Autodesk Inventor part; units mm, degrees
(part 2 of 8)
sketch "1" plane through (0, 0, 0) normal (0, 0, 1) x (1, 0, 0)
  arc A0 (47.7148, 33.2368) -> (47.5352, 33.0572) centre (47.625, 33.147) ccw
  arc A1 (30.9339, 69.4909) -> (31.1879, 69.4909) centre (31.0609, 69.4909) ccw
  line L0 (31.0609, 69.4909) -> (25.4, 63.83)
  arc A2 (25.3102, 63.9198) -> (25.4898, 63.7402) centre (25.4, 63.83) ccw
  line L1 (74.442, 14.6412) -> (67.4932, 21.59)
  arc A3 (46.228, 52.197) -> (46.228, 51.943) centre (46.228, 52.07) ccw
  arc A4 (52.451, 51.943) -> (52.451, 52.197) centre (52.451, 52.07) ccw
  line L2 (46.228, 52.07) -> (52.451, 52.07)
  arc A5 (55.1552, 71.891) -> (55.3348, 72.0706) centre (55.245, 71.9808) ccw
  arc A6 (55.3094, 72.096) -> (55.1298, 71.9164) centre (55.2196, 72.0062) ccw
  line L3 (55.245, 71.9808) -> (55.2196, 72.0062)
  arc A7 (55.118, 54.864) -> (55.372, 54.864) centre (55.245, 54.864) ccw
  arc A8 (55.372, 71.9808) -> (55.118, 71.9808) centre (55.245, 71.9808) ccw
  line L4 (55.245, 54.864) -> (55.245, 71.9808)
  arc A9 (52.3612, 52.1598) -> (52.5408, 51.9802) centre (52.451, 52.07) ccw
  arc A10 (55.3348, 54.7742) -> (55.1552, 54.9538) centre (55.245, 54.864) ccw
  line L5 (52.451, 52.07) -> (55.245, 54.864)
  arc A11 (30.3902, 36.4118) -> (30.5698, 36.2322) centre (30.48, 36.322) ccw
  arc A12 (46.3178, 51.9802) -> (46.1382, 52.1598) centre (46.228, 52.07) ccw
  line L6 (30.48, 36.322) -> (46.228, 52.07)
  arc A13 (31.1507, 69.4011) -> (30.9711, 69.5807) centre (31.0609, 69.4909) ccw
  line L7 (25.4, 36.322) -> (25.4, 63.83)
  arc A14 (25.527, 63.83) -> (25.273, 63.83) centre (25.4, 63.83) ccw
  arc A15 (25.273, 36.322) -> (25.527, 36.322) centre (25.4, 36.322) ccw
  arc A16 (53.9458, 80.9625) -> (53.9458, 81.5975) centre (53.9458, 81.28) ccw
  arc A17 (20.4098, 31.3318) -> (20.2302, 31.1522) centre (20.32, 31.242) ccw
  line L8 (74.442, 9.6412) -> (69.8808, 5.08)
  arc A18 (69.6563, 5.3045) -> (70.1053, 4.8555) centre (69.8808, 5.08) ccw
  arc A19 (74.6665, 9.4167) -> (74.2175, 9.8657) centre (74.442, 9.6412) ccw
  line L9 (57.4105, 5.08) -> (52.8493, 9.6412)
  arc A20 (53.0738, 9.8657) -> (52.6248, 9.4167) centre (52.8493, 9.6412) ccw
  arc A21 (57.186, 4.8555) -> (57.635, 5.3045) centre (57.4105, 5.08) ccw
  line L10 (69.8808, 5.08) -> (57.4105, 5.08)
  arc A22 (57.4105, 5.3975) -> (57.4105, 4.7625) centre (57.4105, 5.08) ccw
  arc A23 (69.8808, 4.7625) -> (69.8808, 5.3975) centre (69.8808, 5.08) ccw
  line L11 (52.8493, 9.6412) -> (48.2881, 5.08)
  arc A24 (48.0636, 5.3045) -> (48.5126, 4.8555) centre (48.2881, 5.08) ccw
  arc A25 (53.0738, 9.4167) -> (52.6248, 9.8657) centre (52.8493, 9.6412) ccw
  line L12 (48.2881, 5.08) -> (35.56, 5.08)
  line L13 (33.6795, 17.8825) -> (33.6795, 15.0888)
  arc A26 (33.5525, 15.0888) -> (33.8065, 15.0888) centre (33.6795, 15.0888) ccw
  arc A27 (33.8065, 17.8825) -> (33.5525, 17.8825) centre (33.6795, 17.8825) ccw
  line L14 (33.6796, 15.0886) -> (33.6795, 15.0888)
  arc A28 (33.7693, 15.1786) -> (33.5897, 14.999) centre (33.6795, 15.0888) ccw
  arc A29 (33.5898, 14.9988) -> (33.7694, 15.1784) centre (33.6796, 15.0886) ccw
  line L15 (33.6795, 17.8825) -> (20.32, 31.242)
  arc A30 (33.5897, 17.7927) -> (33.7693, 17.9723) centre (33.6795, 17.8825) ccw
  line L16 (20.32, 31.242) -> (20.32, 33.782)
  arc A31 (20.447, 33.782) -> (20.193, 33.782) centre (20.32, 33.782) ccw
  arc A32 (20.193, 31.242) -> (20.447, 31.242) centre (20.32, 31.242) ccw
  arc A33 (85.0002, 59.6002) -> (85.1798, 59.7798) centre (85.09, 59.69) ccw
  arc A34 (73.9474, 71.0122) -> (73.7678, 70.8326) centre (73.8576, 70.9224) ccw
  line L17 (85.09, 59.69) -> (73.8576, 70.9224)
  arc A35 (84.963, 50.8) -> (85.217, 50.8) centre (85.09, 50.8) ccw
  arc A36 (85.217, 59.69) -> (84.963, 59.69) centre (85.09, 59.69) ccw
  line L18 (85.09, 50.8) -> (85.09, 59.69)
  arc A37 (73.7306, 70.9224) -> (73.9846, 70.9224) centre (73.8576, 70.9224) ccw
  arc A38 (73.9846, 74.8321) -> (73.7306, 74.8321) centre (73.8576, 74.8321) ccw
  line L19 (73.8576, 70.9224) -> (73.8576, 74.8321)
  arc A39 (61.7944, 42.037) -> (61.7944, 41.783) centre (61.7944, 41.91) ccw
  arc A40 (76.2, 41.783) -> (76.2, 42.037) centre (76.2, 41.91) ccw
  line L20 (61.7944, 41.91) -> (76.2, 41.91)
  arc A41 (76.1102, 41.9998) -> (76.2898, 41.8202) centre (76.2, 41.91) ccw
  arc A42 (85.1798, 50.7102) -> (85.0002, 50.8898) centre (85.09, 50.8) ccw
  line L21 (76.2, 41.91) -> (85.09, 50.8)
  arc A43 (56.1166, 36.4118) -> (56.2962, 36.2322) centre (56.2064, 36.322) ccw
  arc A44 (61.8842, 41.8202) -> (61.7046, 41.9998) centre (61.7944, 41.91) ccw
  line L22 (56.2064, 36.322) -> (61.7944, 41.91)
  line L23 (27.94, 36.322) -> (27.94, 48.2127)
  arc A45 (28.067, 48.2127) -> (27.813, 48.2127) centre (27.94, 48.2127) ccw
  arc A46 (27.813, 36.322) -> (28.067, 36.322) centre (27.94, 36.322) ccw
  line L24 (27.94, 48.2127) -> (31.1842, 51.4569)
  arc A47 (31.274, 51.3671) -> (31.0944, 51.5467) centre (31.1842, 51.4569) ccw
  arc A48 (27.8502, 48.3025) -> (28.0298, 48.1229) centre (27.94, 48.2127) ccw
  arc A49 (69.4833, 56.5839) -> (69.4833, 56.3299) centre (69.4833, 56.4569) ccw
  arc A50 (74.3504, 56.3299) -> (74.3504, 56.5839) centre (74.3504, 56.4569) ccw
  line L25 (69.4833, 56.4569) -> (74.3504, 56.4569)
  arc A51 (50.9994, 36.322) -> (51.2534, 36.322) centre (51.1264, 36.322) ccw
  arc A52 (51.2534, 38.1) -> (50.9994, 38.1) centre (51.1264, 38.1) ccw
  line L26 (51.1264, 36.322) -> (51.1264, 38.1)
  arc A53 (69.5731, 56.3671) -> (69.3935, 56.5467) centre (69.4833, 56.4569) ccw
  arc A54 (51.0366, 38.1898) -> (51.2162, 38.0102) centre (51.1264, 38.1) ccw
  line L27 (69.4833, 56.4569) -> (51.1264, 38.1)
  arc A55 (53.5712, 36.322) -> (53.7617, 36.322) centre (53.6664, 36.322) ccw
  arc A56 (53.7617, 37.2029) -> (53.5712, 37.2029) centre (53.6664, 37.2029) ccw
  line L28 (53.6664, 36.322) -> (53.6664, 37.2029)
  arc A57 (70.5277, 53.9296) -> (70.393, 54.0643) centre (70.4604, 53.997) ccw
  arc A58 (53.599, 37.2703) -> (53.7338, 37.1356) centre (53.6664, 37.203) ccw
  line L29 (70.4604, 53.9969) -> (53.6664, 37.2029)
  arc A59 (76.8104, 53.9017) -> (76.8104, 54.0922) centre (76.8104, 53.9969) ccw
  arc A60 (70.4604, 54.0922) -> (70.4604, 53.9017) centre (70.4604, 53.9969) ccw
  line L30 (76.8104, 53.9969) -> (70.4604, 53.9969)
  arc A61 (79.283, 51.3896) -> (79.4177, 51.5243) centre (79.3503, 51.4569) ccw
  arc A62 (76.8777, 54.0643) -> (76.743, 53.9296) centre (76.8103, 53.997) ccw
  line L31 (79.3504, 51.4569) -> (76.8104, 53.9969)
  arc A63 (47.5352, 36.2848) -> (47.7148, 36.1052) centre (47.625, 36.195) ccw
  arc A64 (72.4798, 60.8702) -> (72.3002, 61.0498) centre (72.39, 60.96) ccw
  line L32 (47.625, 36.195) -> (72.39, 60.96)
  arc A65 (54.1744, 31.623) -> (54.1744, 31.877) centre (54.1744, 31.75) ccw
  arc A66 (49.022, 31.877) -> (49.022, 31.623) centre (49.022, 31.75) ccw
  line L33 (54.1744, 31.75) -> (49.022, 31.75)
  arc A67 (79.4774, 59.0796) -> (79.2234, 59.0796) centre (79.3504, 59.0796) ccw
  arc A68 (79.2234, 56.4569) -> (79.4774, 56.4569) centre (79.3504, 56.4569) ccw
  line L34 (79.3504, 59.0796) -> (79.3504, 56.4569)
  arc A69 (77.5598, 61.0498) -> (77.3802, 60.8702) centre (77.47, 60.96) ccw
  arc A70 (79.2606, 58.9898) -> (79.4402, 59.1694) centre (79.3504, 59.0796) ccw
  line L35 (77.47, 60.96) -> (79.3504, 59.0796)
  arc A71 (72.39, 61.087) -> (72.39, 60.833) centre (72.39, 60.96) ccw
  arc A72 (77.47, 60.833) -> (77.47, 61.087) centre (77.47, 60.96) ccw
  line L36 (72.39, 60.96) -> (77.47, 60.96)
  arc A73 (47.498, 33.147) -> (47.752, 33.147) centre (47.625, 33.147) ccw
  arc A74 (47.752, 36.195) -> (47.498, 36.195) centre (47.625, 36.195) ccw
  line L37 (47.625, 33.147) -> (47.625, 36.195)
  arc A75 (48.9322, 31.6602) -> (49.1118, 31.8398) centre (49.022, 31.75) ccw
  line L38 (27.94, 33.782) -> (27.94, 34.29)
  line L39 (49.022, 31.75) -> (47.625, 33.147)
  arc A76 (56.2962, 33.6922) -> (56.1166, 33.8718) centre (56.2064, 33.782) ccw
  arc A77 (54.0846, 31.8398) -> (54.2642, 31.6602) centre (54.1744, 31.75) ccw
  line L40 (56.2064, 33.782) -> (54.1744, 31.75)
  arc A78 (69.3639, 51.5839) -> (69.3639, 51.3299) centre (69.3639, 51.4569) ccw
  arc A79 (74.3504, 51.3299) -> (74.3504, 51.5839) centre (74.3504, 51.4569) ccw
  line L41 (69.3639, 51.4569) -> (74.3504, 51.4569)
  arc A80 (54.8504, 37.123) -> (55.03, 36.9434) centre (54.9402, 37.0332) ccw
  arc A81 (69.4537, 51.3671) -> (69.2741, 51.5467) centre (69.3639, 51.4569) ccw
  line L42 (54.9402, 37.0332) -> (69.3639, 51.4569)
  arc A82 (54.8132, 35.0558) -> (55.0672, 35.0558) centre (54.9402, 35.0558) ccw
  arc A83 (55.0672, 37.0332) -> (54.8132, 37.0332) centre (54.9402, 37.0332) ccw
  line L43 (54.9402, 35.0558) -> (54.9402, 37.0332)
  arc A84 (53.5766, 33.8718) -> (53.7562, 33.6922) centre (53.6664, 33.782) ccw
  arc A85 (55.03, 34.966) -> (54.8504, 35.1456) centre (54.9402, 35.0558) ccw
  line L44 (53.6664, 33.782) -> (54.9402, 35.0558)
  arc A86 (68.3984, 24.4475) -> (68.3984, 23.8125) centre (68.3984, 24.13) ccw
  arc A87 (75.8336, 23.8125) -> (75.8336, 24.4475) centre (75.8336, 24.13) ccw
  line L45 (68.3984, 24.13) -> (75.8336, 24.13)
  arc A88 (87.5979, 11.9167) -> (88.0469, 12.3657) centre (87.8224, 12.1412) ccw
  arc A89 (76.0581, 24.3545) -> (75.6091, 23.9055) centre (75.8336, 24.13) ccw
  line L46 (87.8224, 12.1412) -> (75.8336, 24.13)
  arc A90 (87.8224, 12.4587) -> (87.8224, 11.8237) centre (87.8224, 12.1412) ccw
  arc A91 (95.4424, 11.8237) -> (95.4424, 12.4587) centre (95.4424, 12.1412) ccw
  line L47 (87.8224, 12.1412) -> (95.4424, 12.1412)
  arc A92 (58.9709, 34.0065) -> (58.5219, 33.5575) centre (58.7464, 33.782) ccw
  arc A93 (68.1739, 23.9055) -> (68.6229, 24.3545) centre (68.3984, 24.13) ccw
  line L48 (58.7464, 33.782) -> (68.3984, 24.13)
  arc A94 (67.1284, 28.2575) -> (67.1284, 27.6225) centre (67.1284, 27.94) ccw
  arc A95 (90.5862, 27.6225) -> (90.5862, 28.2575) centre (90.5862, 27.94) ccw
  line L49 (67.1284, 27.94) -> (90.5862, 27.94)
  arc A96 (90.3616, 28.1645) -> (90.8107, 27.7155) centre (90.5862, 27.94) ccw
  arc A97 (95.6603, 32.5651) -> (95.2113, 33.0141) centre (95.4358, 32.7896) ccw
  line L50 (90.5862, 27.94) -> (95.4358, 32.7896)
  arc A98 (61.5109, 34.0065) -> (61.0619, 33.5575) centre (61.2864, 33.782) ccw
  arc A99 (66.9039, 27.7155) -> (67.3529, 28.1645) centre (67.1284, 27.94) ccw
  line L51 (61.2864, 33.782) -> (67.1284, 27.94)
  arc A100 (87.3125, 49.53) -> (87.9475, 49.53) centre (87.63, 49.53) ccw
  arc A101 (87.9475, 58.1297) -> (87.3125, 58.1297) centre (87.63, 58.1297) ccw
  line L52 (87.63, 49.53) -> (87.63, 58.1297)
  arc A102 (95.1249, 65.9421) -> (95.7599, 65.9421) centre (95.4424, 65.9421) ccw
  arc A103 (95.7599, 74.8321) -> (95.1249, 74.8321) centre (95.4424, 74.8321) ccw
  line L53 (95.4424, 65.9421) -> (95.4424, 74.8321)
  arc A104 (95.6669, 65.7176) -> (95.2179, 66.1666) centre (95.4424, 65.9421) ccw
  arc A105 (87.4055, 58.3542) -> (87.8545, 57.9052) centre (87.63, 58.1297) ccw
  line L54 (95.4424, 65.9421) -> (87.63, 58.1297)
  arc A106 (77.2455, 39.5945) -> (77.6945, 39.1455) centre (77.47, 39.37) ccw
  arc A107 (87.8545, 49.3055) -> (87.4055, 49.7545) centre (87.63, 49.53) ccw
  line L55 (77.47, 39.37) -> (87.63, 49.53)
  arc A108 (61.7944, 39.6875) -> (61.7944, 39.0525) centre (61.7944, 39.37) ccw
  arc A109 (77.47, 39.0525) -> (77.47, 39.6875) centre (77.47, 39.37) ccw
  line L56 (61.7944, 39.37) -> (77.47, 39.37)
  arc A110 (58.5219, 36.5465) -> (58.9709, 36.0975) centre (58.7464, 36.322) ccw
  arc A111 (28.067, 34.29) -> (27.813, 34.29) centre (27.94, 34.29) ccw
  arc A112 (27.813, 33.782) -> (28.067, 33.782) centre (27.94, 33.782) ccw
  line L57 (27.94, 34.29) -> (29.21, 35.56)
  arc A113 (29.2998, 35.4702) -> (29.1202, 35.6498) centre (29.21, 35.56) ccw
  arc A114 (27.8502, 34.3798) -> (28.0298, 34.2002) centre (27.94, 34.29) ccw
  line L58 (29.21, 44.4827) -> (36.1842, 51.4569)
  arc A115 (36.274, 51.3671) -> (36.0944, 51.5467) centre (36.1842, 51.4569) ccw
  arc A116 (29.1202, 44.5725) -> (29.2998, 44.3929) centre (29.21, 44.4827) ccw
  line L59 (29.21, 35.56) -> (29.21, 44.4827)
  arc A117 (29.337, 44.4827) -> (29.083, 44.4827) centre (29.21, 44.4827) ccw
  arc A118 (29.083, 35.56) -> (29.337, 35.56) centre (29.21, 35.56) ccw
  line L60 (12.085, 15.0469) -> (9.0831, 15.0469)
  arc A119 (9.0831, 15.1739) -> (9.0831, 14.9199) centre (9.0831, 15.0469) ccw
  arc A120 (12.085, 14.9199) -> (12.085, 15.1739) centre (12.085, 15.0469) ccw
  line L61 (9.0831, 15.0469) -> (5.08, 19.05)
  arc A121 (5.1698, 19.1398) -> (4.9902, 18.9602) centre (5.08, 19.05) ccw
  arc A122 (8.9933, 14.9571) -> (9.1729, 15.1367) centre (9.0831, 15.0469) ccw
  line L62 (5.08, 19.05) -> (5.08, 26.67)
  arc A123 (5.207, 26.67) -> (4.953, 26.67) centre (5.08, 26.67) ccw
  arc A124 (4.953, 19.05) -> (5.207, 19.05) centre (5.08, 19.05) ccw
  line L63 (7.62, 29.21) -> (5.08, 26.67)
  arc A125 (4.9902, 26.7598) -> (5.1698, 26.5802) centre (5.08, 26.67) ccw
  arc A126 (7.7098, 29.1202) -> (7.5302, 29.2998) centre (7.62, 29.21) ccw
  line L64 (15.24, 33.782) -> (10.668, 29.21)
  arc A127 (10.5782, 29.2998) -> (10.7578, 29.1202) centre (10.668, 29.21) ccw
  arc A128 (15.3298, 33.6922) -> (15.1502, 33.8718) centre (15.24, 33.782) ccw
  line L65 (10.668, 29.21) -> (7.62, 29.21)
  arc A129 (7.62, 29.337) -> (7.62, 29.083) centre (7.62, 29.21) ccw
  arc A130 (10.668, 29.083) -> (10.668, 29.337) centre (10.668, 29.21) ccw
  line L66 (17.78, 33.782) -> (19.05, 35.052)
  arc A131 (19.1398, 34.9622) -> (18.9602, 35.1418) centre (19.05, 35.052) ccw
  arc A132 (21.463, 33.147) -> (21.717, 33.147) centre (21.59, 33.147) ccw
  arc A133 (17.6902, 33.8718) -> (17.8698, 33.6922) centre (17.78, 33.782) ccw
  line L67 (19.05, 59.7948) -> (12.0927, 66.7521)
  arc A134 (12.1825, 66.8419) -> (12.0029, 66.6623) centre (12.0927, 66.7521) ccw
  arc A135 (18.9602, 59.705) -> (19.1398, 59.8846) centre (19.05, 59.7948) ccw
  line L68 (12.0927, 66.7521) -> (12.0927, 71.8321)
  arc A136 (12.2197, 71.8321) -> (11.9657, 71.8321) centre (12.0927, 71.8321) ccw
  arc A137 (11.9657, 66.7521) -> (12.2197, 66.7521) centre (12.0927, 66.7521) ccw
  line L69 (19.05, 35.052) -> (19.05, 59.7948)
  arc A138 (19.177, 59.7948) -> (18.923, 59.7948) centre (19.05, 59.7948) ccw
  arc A139 (18.923, 35.052) -> (19.177, 35.052) centre (19.05, 35.052) ccw
  line L70 (58.7464, 36.322) -> (61.7944, 39.37)
  arc A140 (35.56, 5.3975) -> (35.56, 4.7625) centre (35.56, 5.08) ccw
  arc A141 (48.2881, 4.7625) -> (48.2881, 5.3975) centre (48.2881, 5.08) ccw
  line L71 (35.56, 5.08) -> (30.6796, 9.9604)
  arc A142 (30.9041, 10.1849) -> (30.4551, 9.7359) centre (30.6796, 9.9604) ccw
  arc A143 (35.3355, 4.8555) -> (35.7845, 5.3045) centre (35.56, 5.08) ccw
  line L72 (30.6796, 9.9604) -> (30.6796, 10.0886)
  arc A144 (30.9971, 10.0886) -> (30.3621, 10.0886) centre (30.6796, 10.0886) ccw
  arc A145 (30.3621, 9.9604) -> (30.9971, 9.9604) centre (30.6796, 9.9604) ccw
  line L73 (30.6796, 10.0886) -> (25.671, 5.08)
  arc A146 (25.4465, 5.3045) -> (25.8955, 4.8555) centre (25.671, 5.08) ccw
  arc A147 (30.9041, 9.8641) -> (30.4551, 10.3131) centre (30.6796, 10.0886) ccw
  line L74 (15.0927, 76.8321) -> (19.5406, 81.28)
  arc A148 (19.7651, 81.0555) -> (19.3161, 81.5045) centre (19.5406, 81.28) ccw
  arc A149 (14.8682, 77.0566) -> (15.3172, 76.6076) centre (15.0927, 76.8321) ccw
  line L75 (14.0519, 5.08) -> (9.085, 10.0469)
  arc A150 (9.3095, 10.2714) -> (8.8605, 9.8224) centre (9.085, 10.0469) ccw
  arc A151 (13.8274, 4.8555) -> (14.2764, 5.3045) centre (14.0519, 5.08) ccw
  line L76 (25.671, 5.08) -> (14.0519, 5.08)
  arc A152 (14.0519, 5.3975) -> (14.0519, 4.7625) centre (14.0519, 5.08) ccw
  arc A153 (25.671, 4.7625) -> (25.671, 5.3975) centre (25.671, 5.08) ccw
  line L77 (48.641, 25.4) -> (48.641, 27.559)
  arc A154 (48.9585, 27.559) -> (48.3235, 27.559) centre (48.641, 27.559) ccw
  arc A155 (48.3235, 25.4) -> (48.9585, 25.4) centre (48.641, 25.4) ccw
  line L78 (39.878, 36.322) -> (35.56, 36.322)
  arc A156 (35.56, 36.6395) -> (35.56, 36.0045) centre (35.56, 36.322) ccw
  arc A157 (39.878, 36.0045) -> (39.878, 36.6395) centre (39.878, 36.322) ccw
  line L79 (48.641, 27.559) -> (39.878, 36.322)
  arc A158 (40.1025, 36.5465) -> (39.6535, 36.0975) centre (39.878, 36.322) ccw
  arc A159 (48.4165, 27.3345) -> (48.8655, 27.7835) centre (48.641, 27.559) ccw
  arc A160 (62.0189, 39.1455) -> (61.5699, 39.5945) centre (61.7944, 39.37) ccw
  line L80 (9.085, 10.0469) -> (3.175, 15.9569)
  arc A161 (74.2175, 14.4167) -> (74.6665, 14.8657) centre (74.442, 14.6412) ccw
  line L81 (41.275, 21.59) -> (30.48, 32.385)
  arc A162 (30.7045, 32.6095) -> (30.2555, 32.1605) centre (30.48, 32.385) ccw
  arc A163 (41.0505, 21.3655) -> (41.4995, 21.8145) centre (41.275, 21.59) ccw
  line L82 (30.48, 32.385) -> (30.48, 33.782)
  arc A164 (30.7975, 33.782) -> (30.1625, 33.782) centre (30.48, 33.782) ccw
  arc A165 (30.1625, 32.385) -> (30.7975, 32.385) centre (30.48, 32.385) ccw
  line L83 (67.4932, 21.59) -> (41.275, 21.59)
  arc A166 (41.275, 21.9075) -> (41.275, 21.2725) centre (41.275, 21.59) ccw
  arc A167 (67.4932, 21.2725) -> (67.4932, 21.9075) centre (67.4932, 21.59) ccw
  line L84 (33.02, 36.322) -> (47.5751, 50.8771)
  arc A168 (47.6649, 50.7873) -> (47.4853, 50.9669) centre (47.5751, 50.8771) ccw
  arc A169 (32.9302, 36.4118) -> (33.1098, 36.2322) centre (33.02, 36.322) ccw
  line L85 (47.5751, 50.8771) -> (55.2831, 50.8771)
  arc A170 (55.2831, 50.7501) -> (55.2831, 51.0041) centre (55.2831, 50.8771) ccw
  arc A171 (47.5751, 51.0041) -> (47.5751, 50.7501) centre (47.5751, 50.8771) ccw
  line L86 (52.8493, 14.6412) -> (42.5088, 14.6412)
  arc A172 (42.5088, 14.7682) -> (42.5088, 14.5142) centre (42.5088, 14.6412) ccw
  arc A173 (52.8493, 14.5142) -> (52.8493, 14.7682) centre (52.8493, 14.6412) ccw
  line L87 (42.5088, 14.6412) -> (24.13, 33.02)
  arc A174 (24.2198, 33.1098) -> (24.0402, 32.9302) centre (24.13, 33.02) ccw
  arc A175 (42.419, 14.5514) -> (42.5986, 14.731) centre (42.5088, 14.6412) ccw
  line L88 (24.13, 35.052) -> (22.86, 36.322)
  arc A176 (22.9498, 36.4118) -> (22.7702, 36.2322) centre (22.86, 36.322) ccw
  arc A177 (24.0402, 34.9622) -> (24.2198, 35.1418) centre (24.13, 35.052) ccw
  line L89 (24.13, 33.02) -> (24.13, 35.052)
  arc A178 (24.257, 35.052) -> (24.003, 35.052) centre (24.13, 35.052) ccw
  arc A179 (24.003, 33.02) -> (24.257, 33.02) centre (24.13, 33.02) ccw
  line L90 (57.8493, 14.6412) -> (55.3493, 12.1412)
  arc A180 (55.2595, 12.231) -> (55.4391, 12.0514) centre (55.3493, 12.1412) ccw
  arc A181 (57.9391, 14.5514) -> (57.7595, 14.731) centre (57.8493, 14.6412) ccw
  line L91 (21.59, 35.052) -> (20.32, 36.322)
  arc A182 (20.4098, 36.4118) -> (20.2302, 36.2322) centre (20.32, 36.322) ccw
  arc A183 (21.5002, 34.9622) -> (21.6798, 35.1418) centre (21.59, 35.052) ccw
  line L92 (55.3493, 12.1412) -> (42.5958, 12.1412)
  arc A184 (42.5958, 12.2365) -> (42.5958, 12.046) centre (42.5958, 12.1413) ccw
  arc A185 (55.3493, 12.046) -> (55.3493, 12.2365) centre (55.3493, 12.1413) ccw
  line L93 (42.5958, 12.1412) -> (21.59, 33.147)
  arc A186 (21.6798, 33.2368) -> (21.5002, 33.0572) centre (21.59, 33.147) ccw
  arc A187 (42.506, 12.0514) -> (42.6856, 12.231) centre (42.5958, 12.1412) ccw
  line L94 (21.59, 33.147) -> (21.59, 35.052)
  arc A188 (21.717, 35.052) -> (21.463, 35.052) centre (21.59, 35.052) ccw
  arc A189 (3.3995, 16.1814) -> (2.9505, 15.7324) centre (3.175, 15.9569) ccw
  arc A190 (8.8605, 9.8224) -> (9.3095, 10.2714) centre (9.085, 10.0469) ccw
  line L95 (3.175, 78.105) -> (6.35, 81.28)
  arc A191 (6.5745, 81.0555) -> (6.1255, 81.5045) centre (6.35, 81.28) ccw
  arc A192 (2.9505, 78.3295) -> (3.3995, 77.8805) centre (3.175, 78.105) ccw
  line L96 (6.35, 81.28) -> (10.6448, 81.28)
  arc A193 (10.6448, 80.9625) -> (10.6448, 81.5975) centre (10.6448, 81.28) ccw
  arc A194 (6.35, 81.5975) -> (6.35, 80.9625) centre (6.35, 81.28) ccw
  line L97 (10.6448, 81.28) -> (15.0927, 76.8321)
  arc A195 (14.8682, 76.6076) -> (15.3172, 77.0566) centre (15.0927, 76.8321) ccw
  arc A196 (10.8693, 81.5045) -> (10.4203, 81.0555) centre (10.6448, 81.28) ccw
  line L98 (3.175, 15.9569) -> (3.175, 78.105)
  arc A197 (3.4925, 78.105) -> (2.8575, 78.105) centre (3.175, 78.105) ccw
  arc A198 (2.8575, 15.9569) -> (3.4925, 15.9569) centre (3.175, 15.9569) ccw
  line L99 (53.9458, 81.28) -> (58.2196, 77.0062)
  arc A199 (57.9951, 76.7817) -> (58.4441, 77.2307) centre (58.2196, 77.0062) ccw
  arc A200 (54.1703, 81.5045) -> (53.7213, 81.0555) centre (53.9458, 81.28) ccw
  line L100 (60.8231, 74.4027) -> (60.8231, 58.4171)
  arc A201 (60.5056, 58.4171) -> (61.1406, 58.4171) centre (60.8231, 58.4171) ccw
  arc A202 (61.1406, 74.4027) -> (60.5056, 74.4027) centre (60.8231, 74.4027) ccw
  line L101 (58.2831, 55.8771) -> (60.8231, 58.4171)
  arc A203 (61.0476, 58.1926) -> (60.5986, 58.6416) centre (60.8231, 58.4171) ccw
  arc A204 (58.0586, 56.1016) -> (58.5076, 55.6526) centre (58.2831, 55.8771) ccw
  line L102 (60.8231, 74.4027) -> (58.2196, 77.0062)
  arc A205 (58.4441, 77.2307) -> (57.9951, 76.7817) centre (58.2196, 77.0062) ccw
  arc A206 (60.5986, 74.1782) -> (61.0476, 74.6272) centre (60.8231, 74.4027) ccw
  line L103 (19.5406, 81.28) -> (53.9458, 81.28)
  arc A207 (19.5406, 81.5975) -> (19.5406, 80.9625) centre (19.5406, 81.28) ccw
  line L104 (52.2831, 55.8771) -> (47.2002, 60.96)
  arc A208 (47.4247, 61.1845) -> (46.9757, 60.7355) centre (47.2002, 60.96) ccw
  arc A209 (52.0586, 55.6526) -> (52.5076, 56.1016) centre (52.2831, 55.8771) ccw
  line L105 (47.2002, 60.96) -> (35.56, 60.96)
  arc A210 (35.56, 61.2775) -> (35.56, 60.6425) centre (35.56, 60.96) ccw
  arc A211 (47.2002, 60.6425) -> (47.2002, 61.2775) centre (47.2002, 60.96) ccw
  line L106 (31.1842, 56.4569) -> (31.1842, 56.5842)
  arc A212 (31.5017, 56.5842) -> (30.8667, 56.5842) centre (31.1842, 56.5842) ccw
  arc A213 (30.8667, 56.4569) -> (31.5017, 56.4569) centre (31.1842, 56.4569) ccw
  line L107 (35.56, 60.96) -> (31.1842, 56.5842)
  arc A214 (30.9597, 56.8087) -> (31.4087, 56.3597) centre (31.1842, 56.5842) ccw
  arc A215 (35.7845, 60.7355) -> (35.3355, 61.1845) centre (35.56, 60.96) ccw
  arc A216 (67.7177, 21.8145) -> (67.2687, 21.3655) centre (67.4932, 21.59) ccw
  line L108 (25.4, 33.782) -> (26.67, 35.052)
  arc A217 (26.7598, 34.9622) -> (26.5802, 35.1418) centre (26.67, 35.052) ccw
  arc A218 (25.3102, 33.8718) -> (25.4898, 33.6922) centre (25.4, 33.782) ccw
  line L109 (26.67, 63.021) -> (36.0609, 72.4119)
  arc A219 (36.1507, 72.3221) -> (35.9711, 72.5017) centre (36.0609, 72.4119) ccw
  arc A220 (26.5802, 63.1108) -> (26.7598, 62.9312) centre (26.67, 63.021) ccw
  line L110 (26.67, 35.052) -> (26.67, 63.021)
  arc A221 (26.797, 63.021) -> (26.543, 63.021) centre (26.67, 63.021) ccw
  arc A222 (26.543, 35.052) -> (26.797, 35.052) centre (26.67, 35.052) ccw
  line L111 (31.0609, 69.4909) -> (31.0609, 72.4119)
  arc A223 (31.1879, 72.4119) -> (30.9339, 72.4119) centre (31.0609, 72.4119) ccw
  constraints: 613 point on circle, 224 centre point, 224 end point, 6 point on line
sketch "16" plane through (0, 0, 0) normal (0, 0, 1) x (1, 0, 0)
  line L0 (52.2196, 77.0062) -> (47.9458, 81.28)
  arc A0 (56.4934, 81.5975) -> (56.4934, 80.9625) centre (56.4934, 81.28) ccw
  arc A1 (73.4097, 80.9625) -> (73.4097, 81.5975) centre (73.4097, 81.28) ccw
  arc A2 (7.493, 25.4) -> (7.747, 25.4) centre (7.62, 25.4) ccw
  arc A3 (7.747, 33.782) -> (7.493, 33.782) centre (7.62, 33.782) ccw
  line L1 (7.62, 25.4) -> (7.62, 33.782)
  arc A4 (13.843, 31.75) -> (14.097, 31.75) centre (13.97, 31.75) ccw
  arc A5 (14.097, 35.052) -> (13.843, 35.052) centre (13.97, 35.052) ccw
  line L2 (13.97, 31.75) -> (13.97, 35.052)
  arc A6 (13.8802, 34.9622) -> (14.0598, 35.1418) centre (13.97, 35.052) ccw
  arc A7 (12.7898, 36.4118) -> (12.6102, 36.2322) centre (12.7, 36.322) ccw
  line L3 (13.97, 35.052) -> (12.7, 36.322)
  arc A8 (20.2302, 25.3102) -> (20.4098, 25.4898) centre (20.32, 25.4) ccw
  arc A9 (14.0598, 31.8398) -> (13.8802, 31.6602) centre (13.97, 31.75) ccw
  line L4 (20.32, 25.4) -> (13.97, 31.75)
  arc A10 (22.733, 25.4) -> (22.987, 25.4) centre (22.86, 25.4) ccw
  arc A11 (22.987, 33.782) -> (22.733, 33.782) centre (22.86, 33.782) ccw
  line L5 (22.86, 25.4) -> (22.86, 33.782)
  arc A12 (11.303, 29.21) -> (11.557, 29.21) centre (11.43, 29.21) ccw
  arc A13 (11.557, 35.052) -> (11.303, 35.052) centre (11.43, 35.052) ccw
  line L6 (11.43, 29.21) -> (11.43, 35.052)
  arc A14 (11.3402, 34.9622) -> (11.5198, 35.1418) centre (11.43, 35.052) ccw
  arc A15 (10.2498, 36.4118) -> (10.0702, 36.2322) centre (10.16, 36.322) ccw
  line L7 (11.43, 35.052) -> (10.16, 36.322)
  arc A16 (15.1502, 25.3102) -> (15.3298, 25.4898) centre (15.24, 25.4) ccw
  arc A17 (11.5198, 29.2998) -> (11.3402, 29.1202) centre (11.43, 29.21) ccw
  line L8 (15.24, 25.4) -> (11.43, 29.21)
  arc A18 (12.573, 30.48) -> (12.827, 30.48) centre (12.7, 30.48) ccw
  arc A19 (12.827, 33.782) -> (12.573, 33.782) centre (12.7, 33.782) ccw
  line L9 (12.7, 30.48) -> (12.7, 33.782)
  arc A20 (17.6902, 25.3102) -> (17.8698, 25.4898) centre (17.78, 25.4) ccw
  arc A21 (12.7898, 30.5698) -> (12.6102, 30.3902) centre (12.7, 30.48) ccw
  line L10 (17.78, 25.4) -> (12.7, 30.48)
  arc A22 (10.033, 27.94) -> (10.287, 27.94) centre (10.16, 27.94) ccw
  arc A23 (10.287, 33.782) -> (10.033, 33.782) centre (10.16, 33.782) ccw
  line L11 (10.16, 27.94) -> (10.16, 33.782)
  arc A24 (12.6102, 25.3102) -> (12.7898, 25.4898) centre (12.7, 25.4) ccw
  arc A25 (10.2498, 28.0298) -> (10.0702, 27.8502) centre (10.16, 27.94) ccw
  line L12 (12.7, 25.4) -> (10.16, 27.94)
  line L13 (19.1328, 55.7972) -> (17.0355, 55.7972)
  line L14 (56.4934, 81.28) -> (73.4097, 81.28)
  arc A26 (51.9951, 77.2307) -> (52.4441, 76.7817) centre (52.2196, 77.0062) ccw
  arc A27 (56.7179, 81.0555) -> (56.2689, 81.5045) centre (56.4934, 81.28) ccw
  line L15 (52.2196, 77.0062) -> (56.4934, 81.28)
  arc A28 (30.8364, 77.2394) -> (31.2854, 77.6884) centre (31.0609, 77.4639) ccw
  arc A29 (27.4693, 81.5045) -> (27.0203, 81.0555) centre (27.2448, 81.28) ccw
  line L16 (31.0609, 77.4639) -> (27.2448, 81.28)
  arc A30 (30.7434, 77.4119) -> (31.3784, 77.4119) centre (31.0609, 77.4119) ccw
  arc A31 (31.3784, 77.4639) -> (30.7434, 77.4639) centre (31.0609, 77.4639) ccw
  line L17 (31.0609, 77.4119) -> (31.0609, 77.4639)
  arc A32 (35.2209, 81.28) -> (34.5859, 81.28) centre (34.9034, 81.28) ccw
  arc A33 (34.5859, 81.2544) -> (35.2209, 81.2544) centre (34.9034, 81.2544) ccw
  line L18 (34.9034, 81.28) -> (34.9034, 81.2544)
  arc A34 (30.8364, 77.6364) -> (31.2854, 77.1874) centre (31.0609, 77.4119) ccw
  arc A35 (35.1279, 81.0299) -> (34.6789, 81.4789) centre (34.9034, 81.2544) ccw
  line L19 (31.0609, 77.4119) -> (34.9034, 81.2544)
  arc A36 (44.9875, 21.3655) -> (45.4365, 21.8145) centre (45.212, 21.59) ccw
  arc A37 (33.2445, 34.0065) -> (32.7955, 33.5575) centre (33.02, 33.782) ccw
  line L20 (45.212, 21.59) -> (33.02, 33.782)
  arc A38 (50.8, 21.2725) -> (50.8, 21.9075) centre (50.8, 21.59) ccw
  arc A39 (45.212, 21.9075) -> (45.212, 21.2725) centre (45.212, 21.59) ccw
  arc A40 (53.9455, 24.2865) -> (53.4965, 24.7355) centre (53.721, 24.511) ccw
  arc A41 (50.5755, 21.8145) -> (51.0245, 21.3655) centre (50.8, 21.59) ccw
  line L21 (53.721, 24.511) -> (50.8, 21.59)
  arc A42 (54.0385, 25.4) -> (53.4035, 25.4) centre (53.721, 25.4) ccw
  arc A43 (53.4035, 24.511) -> (54.0385, 24.511) centre (53.721, 24.511) ccw
  line L22 (53.721, 25.4) -> (53.721, 24.511)
  arc A44 (64.3639, 25.6245) -> (64.8129, 25.1755) centre (64.5884, 25.4) ccw
  arc A45 (68.6229, 28.9855) -> (68.1739, 29.4345) centre (68.3984, 29.21) ccw
  line L23 (64.5884, 25.4) -> (68.3984, 29.21)
  arc A46 (56.261, 25.7175) -> (56.261, 25.0825) centre (56.261, 25.4) ccw
  arc A47 (64.5884, 25.0825) -> (64.5884, 25.7175) centre (64.5884, 25.4) ccw
  line L24 (56.261, 25.4) -> (64.5884, 25.4)
  arc A48 (56.261, 25.0825) -> (56.261, 25.7175) centre (56.261, 25.4) ccw
  arc A49 (53.721, 25.7175) -> (53.721, 25.0825) centre (53.721, 25.4) ccw
  line L25 (56.261, 25.4) -> (53.721, 25.4)
  arc A50 (20.0519, 5.3975) -> (20.0519, 4.7625) centre (20.0519, 5.08) ccw
  arc A51 (31.6981, 4.7625) -> (31.6981, 5.3975) centre (31.6981, 5.08) ccw
  line L26 (20.0519, 5.08) -> (31.6981, 5.08)
  arc A52 (15.3095, 10.2714) -> (14.8605, 9.8224) centre (15.085, 10.0469) ccw
  arc A53 (19.8274, 4.8555) -> (20.2764, 5.3045) centre (20.0519, 5.08) ccw
  line L27 (15.085, 10.0469) -> (20.0519, 5.08)
  arc A54 (8.8232, 55.5727) -> (9.2722, 56.0217) centre (9.0477, 55.7972) ccw
  arc A55 (8.0022, 57.2917) -> (7.5532, 56.8427) centre (7.7777, 57.0672) ccw
  line L28 (9.0477, 55.7972) -> (7.7777, 57.0672)
  arc A56 (73.9775, 28.8925) -> (73.9775, 29.5275) centre (73.9775, 29.21) ccw
  arc A57 (68.3984, 29.5275) -> (68.3984, 28.8925) centre (68.3984, 29.21) ccw
  line L29 (73.9775, 29.21) -> (68.3984, 29.21)
  arc A58 (68.1739, 28.9855) -> (68.6229, 29.4345) centre (68.3984, 29.21) ccw
  arc A59 (61.5109, 36.5465) -> (61.0619, 36.0975) centre (61.2864, 36.322) ccw
  line L30 (68.3984, 29.21) -> (61.2864, 36.322)
  arc A60 (80.2345, 35.018) -> (79.7855, 35.467) centre (80.01, 35.2425) ccw
  arc A61 (73.753, 29.4345) -> (74.202, 28.9855) centre (73.9775, 29.21) ccw
  line L31 (80.01, 35.2425) -> (73.9775, 29.21)
  arc A62 (31.3806, 5.08) -> (32.0156, 5.08) centre (31.6981, 5.08) ccw
  arc A63 (32.0156, 5.1071) -> (31.3806, 5.1071) centre (31.6981, 5.1071) ccw
  line L32 (31.6981, 5.08) -> (31.6981, 5.1071)
  arc A64 (36.9041, 9.8641) -> (36.4551, 10.3131) centre (36.6796, 10.0886) ccw
  arc A65 (31.4736, 5.3316) -> (31.9226, 4.8826) centre (31.6981, 5.1071) ccw
  line L33 (36.6796, 10.0886) -> (31.6981, 5.1071)
  arc A66 (41.4637, 4.8555) -> (41.9127, 5.3045) centre (41.6882, 5.08) ccw
  arc A67 (36.9041, 10.3131) -> (36.4551, 9.8641) centre (36.6796, 10.0886) ccw
  line L34 (41.6882, 5.08) -> (36.6796, 10.0886)
  arc A68 (53.2935, 4.7625) -> (53.2935, 5.3975) centre (53.2935, 5.08) ccw
  arc A69 (41.6882, 5.3975) -> (41.6882, 4.7625) centre (41.6882, 5.08) ccw
  line L35 (53.2935, 5.08) -> (41.6882, 5.08)
  arc A70 (58.0738, 9.4113) -> (57.6248, 9.8603) centre (57.8493, 9.6358) ccw
  arc A71 (53.069, 5.3045) -> (53.518, 4.8555) centre (53.2935, 5.08) ccw
  line L36 (57.8493, 9.6358) -> (53.2935, 5.08)
  arc A72 (58.1668, 9.6412) -> (57.5318, 9.6412) centre (57.8493, 9.6412) ccw
  arc A73 (57.5318, 9.6358) -> (58.1668, 9.6358) centre (57.8493, 9.6358) ccw
  line L37 (57.8493, 9.6412) -> (57.8493, 9.6358)
  arc A74 (74.8808, 4.7625) -> (74.8808, 5.3975) centre (74.8808, 5.08) ccw
  line L38 (50.8, 21.59) -> (45.212, 21.59)
  arc A75 (16.811, 55.5727) -> (17.26, 56.0217) centre (17.0355, 55.7972) ccw
  arc A76 (15.2722, 58.0095) -> (14.8232, 57.5605) centre (15.0477, 57.785) ccw
  line L39 (17.0355, 55.7972) -> (15.0477, 57.785)
  arc A77 (17.0355, 55.4797) -> (17.0355, 56.1147) centre (17.0355, 55.7972) ccw
  arc A78 (15.0477, 56.1147) -> (15.0477, 55.4797) centre (15.0477, 55.7972) ccw
  line L40 (17.0355, 55.7972) -> (15.0477, 55.7972)
  arc A79 (19.1328, 55.4797) -> (19.1328, 56.1147) centre (19.1328, 55.7972) ccw
  arc A80 (17.0355, 56.1147) -> (17.0355, 55.4797) centre (17.0355, 55.7972) ccw
  arc A81 (95.4424, 53.3219) -> (95.4424, 54.5919) centre (95.4424, 53.9569) ccw
  arc A82 (35.3355, 39.1455) -> (35.7845, 39.5945) centre (35.56, 39.37) ccw
  arc A83 (19.3573, 56.0217) -> (18.9083, 55.5727) centre (19.1328, 55.7972) ccw
  line L41 (35.56, 39.37) -> (19.1328, 55.7972)
  arc A84 (35.2425, 36.322) -> (35.8775, 36.322) centre (35.56, 36.322) ccw
  arc A85 (35.8775, 39.37) -> (35.2425, 39.37) centre (35.56, 39.37) ccw
  line L42 (35.56, 36.322) -> (35.56, 39.37)
  arc A86 (14.8232, 77.0116) -> (15.2722, 76.5625) centre (15.0477, 76.787) ccw
  arc A87 (15.3172, 76.6076) -> (14.8682, 77.0566) centre (15.0927, 76.8321) ccw
  line L43 (15.0477, 76.7871) -> (15.0927, 76.8321)
  arc A88 (14.7302, 57.785) -> (15.3652, 57.785) centre (15.0477, 57.785) ccw
  arc A89 (15.3652, 76.7871) -> (14.7302, 76.7871) centre (15.0477, 76.7871) ccw
  line L44 (15.0477, 57.785) -> (15.0477, 76.7871)
  arc A90 (14.7302, 55.7972) -> (15.3652, 55.7972) centre (15.0477, 55.7972) ccw
  arc A91 (15.3652, 57.785) -> (14.7302, 57.785) centre (15.0477, 57.785) ccw
  line L45 (15.0477, 55.7972) -> (15.0477, 57.785)
  arc A92 (8.763, 26.67) -> (9.017, 26.67) centre (8.89, 26.67) ccw
  arc A93 (9.017, 35.052) -> (8.763, 35.052) centre (8.89, 35.052) ccw
  line L46 (8.89, 26.67) -> (8.89, 35.052)
  arc A94 (8.8002, 34.9622) -> (8.9798, 35.1418) centre (8.89, 35.052) ccw
  arc A95 (7.7098, 36.4118) -> (7.5302, 36.2322) centre (7.62, 36.322) ccw
  line L47 (8.89, 35.052) -> (7.62, 36.322)
  arc A96 (10.0702, 25.3102) -> (10.2498, 25.4898) centre (10.16, 25.4) ccw
  arc A97 (8.9798, 26.7598) -> (8.8002, 26.5802) centre (8.89, 26.67) ccw
  line L48 (10.16, 25.4) -> (8.89, 26.67)
  arc A98 (11.7302, 39.5143) -> (12.3652, 39.5143) centre (12.0477, 39.5143) ccw
  arc A99 (12.3652, 50.7972) -> (11.7302, 50.7972) centre (12.0477, 50.7972) ccw
  line L49 (12.0477, 39.5143) -> (12.0477, 50.7972)
  arc A100 (15.0155, 36.0975) -> (15.4645, 36.5465) centre (15.24, 36.322) ccw
  arc A101 (12.2722, 39.7388) -> (11.8232, 39.2898) centre (12.0477, 39.5143) ccw
  line L50 (15.24, 36.322) -> (12.0477, 39.5143)
  arc A102 (82.2789, 35.6915) -> (83.177, 34.7935) centre (82.728, 35.2425) ccw
  arc A103 (101.8848, 53.5013) -> (100.9868, 54.3993) centre (101.4358, 53.9503) ccw
  line L51 (82.728, 35.2425) -> (101.4358, 53.9503)
  arc A104 (40.3225, 38.862) -> (40.9575, 38.862) centre (40.64, 38.862) ccw
  arc A105 (40.9575, 72.8328) -> (40.3225, 72.8328) centre (40.64, 72.8328) ccw
  line L52 (40.64, 38.862) -> (40.64, 72.8328)
  arc A106 (40.4155, 72.6083) -> (40.8645, 73.0573) centre (40.64, 72.8328) ccw
  arc A107 (36.2854, 77.6364) -> (35.8364, 77.1874) centre (36.0609, 77.4119) ccw
  line L53 (40.64, 72.8328) -> (36.0609, 77.4119)
  arc A108 (35.3355, 34.0065) -> (35.7845, 33.5575) centre (35.56, 33.782) ccw
  arc A109 (40.8645, 38.6375) -> (40.4155, 39.0865) centre (40.64, 38.862) ccw
  line L54 (35.56, 33.782) -> (40.64, 38.862)
  arc A110 (43.7175, 25.1755) -> (44.1665, 25.6245) centre (43.942, 25.4) ccw
  arc A111 (35.7845, 34.0065) -> (35.3355, 33.5575) centre (35.56, 33.782) ccw
  line L55 (43.942, 25.4) -> (35.56, 33.782)
  arc A112 (46.101, 25.0825) -> (46.101, 25.7175) centre (46.101, 25.4) ccw
  arc A113 (43.942, 25.7175) -> (43.942, 25.0825) centre (43.942, 25.4) ccw
  line L56 (46.101, 25.4) -> (43.942, 25.4)
  arc A114 (62.4105, 5.3975) -> (62.4105, 4.7625) centre (62.4105, 5.08) ccw
  line L57 (74.8808, 5.08) -> (62.4105, 5.08)
  arc A115 (62.186, 4.8555) -> (62.635, 5.3045) centre (62.4105, 5.08) ccw
  arc A116 (58.0738, 9.8657) -> (57.6248, 9.4167) centre (57.8493, 9.6412) ccw
  line L58 (62.4105, 5.08) -> (57.8493, 9.6412)
  arc A117 (79.6665, 9.4167) -> (79.2175, 9.8657) centre (79.442, 9.6412) ccw
  arc A118 (74.6563, 5.3045) -> (75.1053, 4.8555) centre (74.8808, 5.08) ccw
  line L59 (79.442, 9.6412) -> (74.8808, 5.08)
  arc A119 (94.3812, 4.7625) -> (94.3812, 5.3975) centre (94.3812, 5.08) ccw
  arc A120 (84.0032, 5.3975) -> (84.0032, 4.7625) centre (84.0032, 5.08) ccw
  line L60 (94.3812, 5.08) -> (84.0032, 5.08)
  arc A121 (83.7787, 4.8555) -> (84.2277, 5.3045) centre (84.0032, 5.08) ccw
  arc A122 (79.6665, 9.8657) -> (79.2175, 9.4167) centre (79.442, 9.6412) ccw
  line L61 (84.0032, 5.08) -> (79.442, 9.6412)
  arc A123 (80.01, 35.8775) -> (80.01, 34.6075) centre (80.01, 35.2425) ccw
  arc A124 (82.728, 34.6075) -> (82.728, 35.8775) centre (82.728, 35.2425) ccw
  line L62 (80.01, 35.2425) -> (82.728, 35.2425)
  arc A125 (101.6669, 11.9167) -> (101.2179, 12.3657) centre (101.4424, 12.1412) ccw
  arc A126 (94.1567, 5.3045) -> (94.6057, 4.8555) centre (94.3812, 5.08) ccw
  arc A127 (101.1249, 53.9569) -> (101.7599, 53.9569) centre (101.4424, 53.9569) ccw
  line L63 (101.4424, 12.1412) -> (94.3812, 5.08)
  arc A128 (101.7599, 32.783) -> (101.1249, 32.783) centre (101.4424, 32.783) ccw
  arc A129 (101.1249, 12.1412) -> (101.7599, 12.1412) centre (101.4424, 12.1412) ccw
  line L64 (101.4424, 32.783) -> (101.4424, 12.1412)
  arc A130 (101.6603, 33.0141) -> (101.2113, 32.5651) centre (101.4358, 32.7896) ccw
  arc A131 (101.2179, 32.5585) -> (101.6669, 33.0076) centre (101.4424, 32.7831) ccw
  line L65 (101.4358, 32.7896) -> (101.4424, 32.783)
  arc A132 (13.5406, 81.5975) -> (13.5406, 80.9625) centre (13.5406, 81.28) ccw
  arc A133 (27.2448, 80.9625) -> (27.2448, 81.5975) centre (27.2448, 81.28) ccw
  line L66 (13.5406, 81.28) -> (27.2448, 81.28)
  arc A134 (73.6342, 81.5045) -> (73.1851, 81.0555) centre (73.4096, 81.28) ccw
  arc A135 (79.633, 74.6076) -> (80.0821, 75.0566) centre (79.8576, 74.8321) ccw
  line L67 (73.4097, 81.28) -> (79.8576, 74.8321)
  arc A136 (94.9945, 80.9625) -> (94.9945, 81.5975) centre (94.9945, 81.28) ccw
  arc A137 (86.3055, 81.5975) -> (86.3055, 80.9625) centre (86.3055, 81.28) ccw
  line L68 (94.9945, 81.28) -> (86.3055, 81.28)
  arc A138 (86.53, 81.0555) -> (86.0809, 81.5045) centre (86.3055, 81.28) ccw
  arc A139 (79.633, 75.0566) -> (80.0821, 74.6076) centre (79.8576, 74.8321) ccw
  line L69 (86.3055, 81.28) -> (79.8576, 74.8321)
  arc A140 (101.2179, 74.6076) -> (101.6669, 75.0566) centre (101.4424, 74.8321) ccw
  arc A141 (95.219, 81.5045) -> (94.77, 81.0555) centre (94.9945, 81.28) ccw
  line L70 (101.4424, 74.8321) -> (94.9945, 81.28)
  arc A142 (110.49, -0.127) -> (110.49, 0.127) centre (110.49, 0) ccw
  arc A143 (0, 0.127) -> (0, -0.127) centre (0, 0) ccw
  line L71 (110.49, 0) -> (0, 0)
  arc A144 (110.617, 86.36) -> (110.363, 86.36) centre (110.49, 86.36) ccw
  arc A145 (110.363, 0) -> (110.617, 0) centre (110.49, 0) ccw
  line L72 (110.49, 86.36) -> (110.49, 0)
  arc A146 (0, 86.487) -> (0, 86.233) centre (0, 86.36) ccw
  arc A147 (110.49, 86.233) -> (110.49, 86.487) centre (110.49, 86.36) ccw
  line L73 (0, 86.36) -> (110.49, 86.36)
  arc A148 (-0.127, 0) -> (0.127, 0) centre (0, 0) ccw
  arc A149 (0.127, 86.36) -> (-0.127, 86.36) centre (0, 86.36) ccw
  arc A150 (101.7599, 74.8321) -> (101.1249, 74.8321) centre (101.4424, 74.8321) ccw
  line L74 (0, 0) -> (0, 86.36)
  arc A151 (94.1442, 53.5079) -> (93.2462, 54.4059) centre (93.6952, 53.9569) ccw
  arc A152 (74.5318, 35.6915) -> (75.4298, 34.7935) centre (74.9808, 35.2425) ccw
  line L75 (93.6952, 53.9569) -> (74.9808, 35.2425)
  arc A153 (93.6952, 54.5919) -> (93.6952, 53.3219) centre (93.6952, 53.9569) ccw
  line L76 (95.4424, 53.9569) -> (93.6952, 53.9569)
  arc A154 (50.8089, 25.4546) -> (51.4439, 25.4546) centre (51.1264, 25.4546) ccw
  arc A155 (51.4439, 33.782) -> (50.8089, 33.782) centre (51.1264, 33.782) ccw
  line L77 (51.1264, 25.4546) -> (51.1264, 33.782)
  arc A156 (50.9565, 25.1755) -> (51.4055, 25.6245) centre (51.181, 25.4) ccw
  arc A157 (51.3509, 25.6791) -> (50.9019, 25.2301) centre (51.1264, 25.4546) ccw
  line L78 (51.181, 25.4) -> (51.1264, 25.4546)
  arc A158 (46.7655, 38.3245) -> (47.2145, 37.8755) centre (46.99, 38.1) ccw
  arc A159 (49.7545, 40.4155) -> (49.3055, 40.8645) centre (49.53, 40.64) ccw
  line L79 (46.99, 38.1) -> (49.53, 40.64)
  arc A160 (46.6725, 35.56) -> (47.3075, 35.56) centre (46.99, 35.56) ccw
  arc A161 (47.3075, 38.1) -> (46.6725, 38.1) centre (46.99, 38.1) ccw
  line L80 (46.99, 35.56) -> (46.99, 38.1)
  arc A162 (48.5435, 33.5575) -> (48.9925, 34.0065) centre (48.768, 33.782) ccw
  arc A163 (47.2145, 35.7845) -> (46.7655, 35.3355) centre (46.99, 35.56) ccw
  line L81 (48.768, 33.782) -> (46.99, 35.56)
  arc A164 (51.1264, 33.4645) -> (51.1264, 34.0995) centre (51.1264, 33.782) ccw
  arc A165 (48.768, 34.0995) -> (48.768, 33.4645) centre (48.768, 33.782) ccw
  line L82 (101.4424, 53.9569) -> (101.4424, 74.8321)
  arc A166 (101.1183, 32.7896) -> (101.7533, 32.7896) centre (101.4358, 32.7896) ccw
  arc A167 (101.7533, 53.9503) -> (101.1183, 53.9503) centre (101.4358, 53.9503) ccw
  line L83 (101.4358, 32.7896) -> (101.4358, 53.9503)
  arc A168 (101.2113, 54.1748) -> (101.6603, 53.7258) centre (101.4358, 53.9503) ccw
  arc A169 (101.6669, 53.7324) -> (101.2179, 54.1814) centre (101.4424, 53.9569) ccw
  line L84 (101.4358, 53.9503) -> (101.4424, 53.9569)
  arc A170 (8.8682, 77.0566) -> (9.3172, 76.6076) centre (9.0927, 76.8321) ccw
  arc A171 (13.7651, 81.0555) -> (13.3161, 81.5045) centre (13.5406, 81.28) ccw
  line L85 (9.0927, 76.8321) -> (13.5406, 81.28)
  arc A172 (7.4602, 57.0672) -> (8.0952, 57.0672) centre (7.7777, 57.0672) ccw
  arc A173 (8.0952, 75.5171) -> (7.4602, 75.5171) centre (7.7777, 75.5171) ccw
  line L86 (7.7777, 57.0672) -> (7.7777, 75.5171)
  arc A174 (7.5532, 75.7416) -> (8.0022, 75.2925) centre (7.7777, 75.5171) ccw
  arc A175 (9.3172, 76.6076) -> (8.8682, 77.0566) centre (9.0927, 76.8321) ccw
  line L87 (7.7777, 75.5171) -> (9.0927, 76.8321)
  arc A176 (51.2671, 75.7362) -> (50.6321, 75.7362) centre (50.9496, 75.7362) ccw
  arc A177 (50.6321, 57.2106) -> (51.2671, 57.2106) centre (50.9496, 57.2106) ccw
  line L88 (51.1264, 33.782) -> (48.768, 33.782)
  arc A178 (49.53, 40.9575) -> (49.53, 40.3225) centre (49.53, 40.64) ccw
  arc A179 (69.5833, 40.3225) -> (69.5833, 40.9575) centre (69.5833, 40.64) ccw
  line L89 (49.53, 40.64) -> (69.5833, 40.64)
  arc A180 (74.7563, 35.018) -> (75.2053, 35.467) centre (74.9808, 35.2425) ccw
  arc A181 (69.8078, 40.8645) -> (69.3588, 40.4155) centre (69.5833, 40.64) ccw
  line L90 (74.9808, 35.2425) -> (69.5833, 40.64)
  arc A182 (20.2105, 61.2775) -> (20.2105, 60.6425) centre (20.2105, 60.96) ccw
  arc A183 (32.9511, 60.6425) -> (32.9511, 61.2775) centre (32.9511, 60.96) ccw
  line L91 (20.2105, 60.96) -> (32.9511, 60.96)
  arc A184 (35.9597, 57.5024) -> (36.4087, 57.9514) centre (36.1842, 57.7269) ccw
  arc A185 (33.1756, 61.1845) -> (32.7266, 60.7355) centre (32.9511, 60.96) ccw
  line L92 (36.1842, 57.7269) -> (32.9511, 60.96)
  arc A186 (36.5017, 57.7269) -> (35.8667, 57.7269) centre (36.1842, 57.7269) ccw
  arc A187 (35.8667, 56.4569) -> (36.5017, 56.4569) centre (36.1842, 56.4569) ccw
  line L93 (36.1842, 57.7269) -> (36.1842, 56.4569)
  arc A188 (14.8232, 56.0217) -> (15.2722, 55.5727) centre (15.0477, 55.7972) ccw
  arc A189 (20.435, 60.7355) -> (19.986, 61.1845) centre (20.2105, 60.96) ccw
  line L94 (15.0477, 55.7972) -> (20.2105, 60.96)
  line L95 (50.9496, 75.7362) -> (50.9496, 57.2106)
  arc A190 (50.7251, 75.9607) -> (51.1741, 75.5117) centre (50.9496, 75.7362) ccw
  arc A191 (52.4441, 76.7817) -> (51.9951, 77.2307) centre (52.2196, 77.0062) ccw
  line L96 (50.9496, 75.7362) -> (52.2196, 77.0062)
  arc A192 (52.0586, 55.6526) -> (52.5076, 56.1016) centre (52.2831, 55.8771) ccw
  arc A193 (51.1741, 57.4351) -> (50.7251, 56.9861) centre (50.9496, 57.2106) ccw
  line L97 (52.2831, 55.8771) -> (50.9496, 57.2106)
  arc A194 (47.9458, 80.9625) -> (47.9458, 81.5975) centre (47.9458, 81.28) ccw
  arc A195 (34.9034, 81.5975) -> (34.9034, 80.9625) centre (34.9034, 81.28) ccw
  line L98 (47.9458, 81.28) -> (34.9034, 81.28)
  arc A196 (51.9951, 76.7817) -> (52.4441, 77.2307) centre (52.2196, 77.0062) ccw
  arc A197 (48.1703, 81.5045) -> (47.7213, 81.0555) centre (47.9458, 81.28) ccw
  constraints: 552 point on circle, 198 centre point, 198 end point, 34 point on line